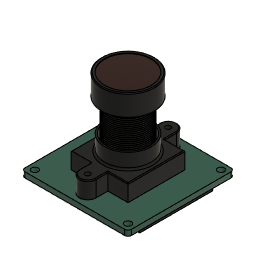
raspberry_pi_cam_8mp_m12_lens (Autodesk Fusion 360 design; units mm, degrees)
Autodesk Fusion 360 part; units mm, degrees
sketch "Sketch1" plane through (0, 0, 0) normal (0, 0, 1) x (1, 0, 0) in component "Board"
  line L0 (15, -16) -> (-15, -16)
  line L1 (-16, -15) -> (-16, 15)
  line L2 (-15, 16) -> (15, 16)
  line L3 (16, 15) -> (16, -15)
  line L4 (16, -16) -> (-16, 16) construction
  line L5 (-16, -16) -> (16, 16) construction
  arc A0 (-15, 16) -> (-16, 15) centre (-15, 15) ccw
  arc A1 (16, 15) -> (15, 16) centre (15, 15) ccw
  arc A2 (15, -16) -> (16, -15) centre (15, -15) ccw
  arc A3 (-16, -15) -> (-15, -16) centre (-15, -15) ccw
  circle A4 centre (-14, 14) radius 1
  circle A5 centre (14, 14) radius 1
  circle A6 centre (-14, -14) radius 1
  circle A7 centre (14, -14) radius 1
  dimension "d1" = 32
  dimension "d2" = 32
  dimension "d3" = 1
  dimension "d4" = 2
  dimension "d5" = 2
  dimension "d8" = 28
  dimension "d9" = -28
  constraint horizontal L0
  constraint perpendicular L0 L1
  constraint parallel L0 L2
  constraint parallel L1 L3
  constraint coincident L4 origin
  constraint coincident L5 origin
  constraint coincident L4.end L2
  constraint coincident L4.end L1
  constraint tangent L2 A0
  constraint tangent L1 A0
  constraint coincident L5.end L2
  constraint coincident L5.end L3
  constraint tangent L2 A1
  constraint tangent L3 A1
  constraint equal A0 A1
  constraint coincident L4.start L3
  constraint coincident L4.start L0
  constraint tangent L3 A2
  constraint tangent L0 A2
  constraint equal A0 A2
  constraint coincident L5.start L0
  constraint coincident L5.start L1
  constraint tangent L0 A3
  constraint tangent L1 A3
  constraint equal A0 A3
  constraint coincident L4 A4.centre
  measures "d1" distance of L4.end L5.end
  measures "d2" distance of L5.start L4.end
  measures "d3" radius of A0
  measures "d4" diameter of A4
  measures "d5" distance of L2 A4.centre
extrude "Extrude1" add sketch "Sketch1" along normal blind 1.6 makes body 1 in component "Board"
sketch "Sketch1 (2)" plane through (0, 0, 1.6) normal (0, 0, 1) x (-1, 0, 0) in component "Camera"
  circle A0 centre (14, -14) radius 1
  circle A1 centre (-14, 14) radius 1
  circle A2 centre (14, 14) radius 1
  circle A3 centre (-14, -14) radius 1
  arc A4 (15, -16) -> (16, -15) centre (15, -15) ccw
  line L0 (16, -15) -> (16, 15)
  arc A5 (16, 15) -> (15, 16) centre (15, 15) ccw
  line L1 (15, 16) -> (-15, 16)
  arc A6 (-15, 16) -> (-16, 15) centre (-15, 15) ccw
  line L2 (-16, 15) -> (-16, -15)
  arc A7 (-16, -15) -> (-15, -16) centre (-15, -15) ccw
  line L3 (-15, -16) -> (15, -16)
  line L4 (-8.55, 8.55) -> (8.55, 8.55)
  line L5 (8.55, 8.55) -> (8.55, -8.55)
  line L6 (8.55, -8.55) -> (-8.55, -8.55)
  line L7 (-8.55, -8.55) -> (-8.55, 8.55)
  line L8 (-8.55, 8.55) -> (8.55, -8.55) construction
  line L9 (8.55, 8.55) -> (-8.55, -8.55) construction
  line L10 (2.5, -12.1) -> (2.5, 12.1)
  arc A8 (2.5, 12.1) -> (-2.5, 12.1) centre (0, 12.1) ccw
  line L11 (-2.5, 12.1) -> (-2.5, -12.1)
  arc A9 (-2.5, -12.1) -> (2.5, -12.1) centre (0, -12.1) ccw
  line L12 (0, -12.1) -> (0, 12.1) construction
  circle A10 centre (0, -12.1) radius 0.75
  line L13 (8.55, 0) -> (-8.55, 0) construction
  circle A11 centre (0, 12.1) radius 0.75
  circle A12 centre (0, 0) radius 7
  circle A13 centre (0, 0) radius 6.5
  dimension "d12" = 17.1
  dimension "d13" = 17.1
  dimension "d14" = 5
  dimension "d15" = 24.2
  dimension "d16" = 1.5
  dimension "d17" = 14
  dimension "d18" = -0.5
  constraint horizontal L4
  constraint perpendicular L4 L5
  constraint parallel L4 L6
  constraint parallel L5 L7
  constraint coincident L8 A12.centre
  constraint coincident L9 A12.centre
  constraint coincident A12.centre A13.centre
  constraint tangent L10 A8
  constraint tangent A8 L11
  constraint parallel L10 L11
  constraint tangent L11 A9
  constraint tangent L10 A9
  constraint parallel L0 L12
  constraint midpoint L12 A12.centre
  constraint concentric A9 A10
  constraint midpoint L5 L13.start
  constraint midpoint L7 L13.end
  constraint symmetric A10 L13 A11
  measures "d12" distance of L5.end L6.end
  measures "d13" distance of L4.end L5.end
  measures "d14" diameter of A8
  measures "d15" distance of A9.centre A8.centre
  measures "d16" diameter of A10
  measures "d17" diameter of A12
extrude "Extrude1'" add sketch "Sketch1 (2)" along normal blind 5 separate body contours L4 L6 L7 L11 A12 | L4 L10 A8 L11 | L4 L10 L11 A12 | L4 L5 L6 L10 A12 | L10 L11 A12 A13 | L11 A12 A13 | L6 L10 L11 A12 | L6 L10 L11 A9 | L10 A12 A13 | L10 L11 A13 | L11 A13 | L10 L11 A12 A13 | L10 A13 makes body 2 in component "Camera"
extrude "Extrude2" add sketch "Sketch1 (2)" along normal blind 4.5 from surface at 5 contours L10 L11 A12 A13 | L11 A12 A13 | L10 A12 A13 | L10 L11 A12 A13 bodies 2 in component "Camera"
sketch "Sketch2" plane through (0, 0, 6.6) normal (0, 0, 1) x (-1, 0, 0) in component "Camera"
  circle A0 centre (0, 0) radius 6.5
  circle A1 centre (0, 0) radius 6
  circle A2 centre (0, 0) radius 7.9
  dimension "d24" = 12
  dimension "d25" = 15.8
  constraint coincident A0.centre A1.centre
  constraint concentric A1 A2
  measures "d24" diameter of A1
  measures "d25" diameter of A2
extrude "Extrude3" add sketch "Sketch2" along normal blind 14 separate body contours A1 makes body 3 in component "Camera"
extrude "Extrude4" add sketch "Sketch2" along normal blind 6.5 from surface at 14 separate body contours A0 | A2 makes body 4 in component "Camera"
sketch "Sketch3" plane through (0, 0, 27.1) normal (0, 0, 1) x (-1, 0, 0) in component "Camera"
  circle A0 centre (0, 0) radius 6
  circle A1 centre (0, 0) radius 7.9
  circle A2 centre (0, 0) radius 7
  dimension "d31" = 1
extrude "Extrude5" cut sketch "Sketch3" against normal blind 1.5 contours A2 bodies 3 2 4 in component "Camera"
extrude "Extrude6" add sketch "Sketch3" against normal up to surface (1.5 mm away) separate body contours A0 | A2 makes body 5 in component "Camera"
copy_body "Body->Comp1" bodies 5 removing the originals makes body 6 in component "Lens"
sketch "Sketch1 (3)" plane through (0, 0, 0) normal (0, 0, -1) x (1, 0, 0) in component "Ribbon Connector"
  circle A0 centre (-14, -14) radius 1
  circle A1 centre (14, 14) radius 1
  circle A2 centre (-14, 14) radius 1
  circle A3 centre (14, -14) radius 1
  arc A4 (-16, -15) -> (-15, -16) centre (-15, -15) ccw
  line L0 (-15, -16) -> (15, -16)
  arc A5 (15, -16) -> (16, -15) centre (15, -15) ccw
  line L1 (16, -15) -> (16, 15)
  arc A6 (16, 15) -> (15, 16) centre (15, 15) ccw
  line L2 (15, 16) -> (-15, 16)
  arc A7 (-15, 16) -> (-16, 15) centre (-15, 15) ccw
  line L3 (-16, 15) -> (-16, -15)
  line L4 (16, 0) -> (-16, 0) construction
  line L5 (0, 16) -> (0, -16) construction
  line L6 (9, -11) -> (14.5, -11)
  line L7 (14.5, -11) -> (14.5, 11)
  line L8 (14.5, 11) -> (9, 11)
  line L9 (9, 11) -> (9, -11)
  line L10 (9, -11) -> (14.5, 11) construction
  line L11 (14.5, -11) -> (9, 11) construction
  line L12 (9.5, -10.5) -> (14, -10.5)
  line L13 (14, -10.5) -> (14, 10.5)
  line L14 (14, 10.5) -> (9.5, 10.5)
  line L15 (9.5, 10.5) -> (9, 10.5)
  line L16 (9.5, -10.5) -> (9, -10.5)
  line L17 (10.5, 11) -> (10.5, 10.5)
  line L18 (10.5, -11) -> (10.5, -10.5)
  point P0 (11.75, 0)
  dimension "d36" = 5.5
  dimension "d37" = 22
  dimension "d38" = 1.5
  dimension "d40" = 4
  constraint midpoint L1 L4.start
  constraint midpoint L3 L4.end
  constraint midpoint L2 L5.start
  constraint midpoint L0 L5.end
  constraint horizontal L6
  constraint perpendicular L6 L7
  constraint parallel L6 L8
  constraint parallel L7 L9
  constraint coincident L10 P0
  constraint coincident L11 P0
  constraint coincident L4 P0
  constraint coincident L9 L15.end
  constraint perpendicular L9 L15
  constraint coincident L9 L16.end
  constraint perpendicular L9 L16
  constraint coincident L8 L17.start
  constraint coincident L14 L17.end
  constraint perpendicular L14 L17
  constraint symmetric L4 L17.start L18.start
  constraint symmetric L4 L17.end L18.end
  measures "d36" distance of L7.end L8.end
  measures "d37" distance of L6.end L7.end
  measures "d38" distance of L1 L7
  measures "d40" distance of L7 L17
extrude "Extrude1''" add sketch "Sketch1 (3)" along normal blind 2.1 separate body contours L6 L9 L12 L16 L18 | L9 L12 L13 L14 L15 L16 | L8 L9 L14 L15 L17 makes body 7 in component "Ribbon Connector"
sketch "Sketch2 (2)" plane through (14, 0, 0) normal (1, 0, 0) x (0, 1, 0) in component "Ribbon Connector"
  line L0 (10.5, 0) -> (-10.5, 0)
  line L1 (-10.5, 0) -> (-10.5, -2.1)
  line L2 (-10.5, -2.1) -> (10.5, -2.1)
  line L3 (10.5, -2.1) -> (10.5, 0)
  line L4 (8, -0.9) -> (-8, -0.9)
  line L5 (-8, -0.9) -> (-8, -0.5)
  line L6 (-8, -0.5) -> (8, -0.5)
  line L7 (8, -0.5) -> (8, -0.9)
  line L8 (11, 0) -> (-11, 0)
  line L9 (10.5, 0) -> (10.5, -2.1)
  dimension "d43" = 2.5
  dimension "d44" = 16
  dimension "d45" = 0.5
  dimension "d46" = 1.2
  constraint horizontal L4
  constraint vertical L5
  constraint horizontal L6
  constraint vertical L7
  constraint coincident L0.start L3.end
  constraint coincident L2.end L3.start
  measures "d43" distance of L3 L7
  measures "d44" distance of L5 L7
  measures "d45" distance of L6 L8
  measures "d46" distance of L2 L4
extrude "Extrude2'" add sketch "Sketch1 (3)" along normal up to surface (2.1 mm away) separate body contours L6 L7 L8 L12 L13 L14 L17 L18 makes body 8 in component "Ribbon Connector"
extrude "Extrude3'" cut sketch "Sketch2 (2)" along normal mid plane 7 contours L4 L5 L6 L7 bodies 7 8 in component "Ribbon Connector"
move_face "OffsetFaces1" offset -0.5 1 faces at (14.3333, 2.6667, -0.5) on bodies 8 in component "Ribbon Connector"
fillet "Fillet1" radius 1 4 edges at (10.5, -10.75, -2.1) (10.5, -10.75, 0) (10.5, 10.75, 0) (10.5, 10.75, -2.1) on bodies 8 in component "Ribbon Connector"
thread "Thread1" "ISO Metric profile 12.0 M12x0.5 6g" major diameter 11.927 minor diameter 11.348 pitch 0.5 angle 60 modelled right hand crest width 0.0671 on face at (-5.9702, 0.5974, 15.9333) crest through (-5.9635, 0, 6.475) on bodies 3 in component "Camera"
combine "Combine1" operation add target body 3 tool bodies 4 2 makes body 9 at (-7.8607, 0.7866, 22.7667) in component "Camera"
move_face "OffsetFaces1'" offset 0.25 1 faces at (-5.9702, 0.5974, 22.2667) on bodies 9 in component "Camera"
combine "Combine2" operation add target body 9 tool bodies 3 in component "Camera"
move_face "OffsetFaces1''" offset -0.2 1 faces at (-2.7352, 2.3268, 27.1) on bodies 6 in component "Lens"
chamfer "Chamfer1" distance 0.5 angle 45 1 edges at (14, 0, -0.5) on bodies 7 in component "Ribbon Connector"
fillet "Fillet1'" radius 0.5 1 edges at (6.5263, -2.5313, 6.6) on bodies 9 in component "Camera"
fillet "Fillet1'" radius 0.25 11 edges at (2.5, 10.325, 6.6) (0, 14.6, 6.6) (-2.5, 10.325, 6.6) (5.525, 8.55, 6.6) (8.55, 0, 6.6) (5.525, -8.55, 6.6) (-2.5, -10.325, 6.6) (0, -14.6, 6.6) (2.5, -10.325, 6.6) (-8.55, 0, 6.6) (-5.525, 8.55, 6.6) on bodies 9 in component "Camera"
fillet "Fillet1'" radius 0.25 2 edges at (7.3654, -2.8568, 20.6) (7.3654, 2.8568, 27.1) on bodies 9 in component "Camera"
component "Board" placed x (1, 0, 0) y (0, 1, 0) z (0, 0, 1) at (0, 0, 0)
component "Camera" placed x (1, 0, 0) y (0, 1, 0) z (0, 0, 1) at (0, 0, 0)
component "Ribbon Connector" placed x (1, 0, 0) y (0, 1, 0) z (0, 0, 1) at (0, 0, 0)
component "Lens" placed x (1, 0, 0) y (0, 1, 0) z (0, 0, 1) at (0, 0, 0) in component "Camera"
